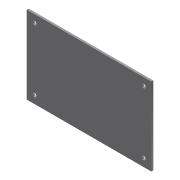
# Autodesk Inventor part: DriveTrain_MotorMount
Saved by Autodesk Inventor 2012 (Build 160160000, 160)
## iProperties
Created: 2012-01-08
Part Number: DriveTrain_MotorMount
Material: Default
Document SubType Name: Modeling
Designer: JesseK
Density: 1 g/cm^3
Author: JesseK
Autodesk Inventor part; units mm, degrees
ref_plane "YZ Plane" through (0, 0, 0) normal (1, 0, 0) x (0, 1, 0)
ref_plane "XZ Plane" through (0, 0, 0) normal (0, 1, 0) x (-1, 0, 0)
ref_plane "XY Plane" through (0, 0, 0) normal (0, 0, 1) x (1, 0, 0)
sketch "Sketch1" plane through (0, 0, 0) normal (0, 0, 1) x (1, 0, 0)
  line L0 (0, 0) -> (203.2, 0)
  line L1 (203.2, 0) -> (203.2, 127)
  line L2 (203.2, 127) -> (0, 127)
  line L3 (0, 127) -> (0, 0)
  circle A0 centre (12.7, 114.3) radius 3.175
  circle A1 centre (12.7, 12.7) radius 3.175
  circle A2 centre (190.5, 114.3) radius 3.175
  circle A3 centre (190.5, 12.7) radius 3.175
  dimension "d0" = 127
  dimension "d1" = 203.2
  dimension "d4" = 12.7
  dimension "d5" = 12.7
  dimension "d6" = 12.7
  dimension "d7" = 12.7
  dimension "d8" = 12.7
  dimension "d9" = 12.7
  dimension "d10" = 12.7
  dimension "d11" = 6.35
  dimension "d12" = 6.35
  dimension "d13" = 12.7
  dimension "d14" = 6.35
  dimension "d15" = 6.35
  constraints: 8 end point, 4 centre point, 2 parallel, 1 horizontal, 1 perpendicular
  measures "d0" distance of L2.end L0.start
  measures "d1" distance of L0.start L0.end
  measures "d4" distance from line of L3 A0.centre
  measures "d5" distance from line of L2 A0.centre
  measures "d6" distance from line of L2 A2.centre
  measures "d7" distance from line of L0 A3.centre
  measures "d8" distance from line of L1 A3.centre
  measures "d9" distance from line of L0 A1.centre
  measures "d10" distance from line of L3 A1.centre
  measures "d11" diameter of A1
  measures "d12" diameter of A0
  measures "d13" distance from line of L1 A2.centre
  measures "d14" diameter of A2
  measures "d15" diameter of A3
extrude "Extrusion2" add sketch "Sketch1" along normal blind 3.175
body "Solid2"
